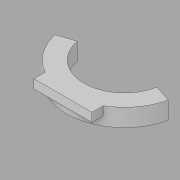
# Autodesk Inventor part: g_jaws
Saved by Autodesk Inventor 2019 (Build 230136000, 136)
## iProperties
Created: 2021-11-03
Part Number: g_jaws
Material: Generic
Document SubType Name: Modeling
Designer: Mohamed
Density: 1 g/cm^3
Appearance: Default
Author: Mohamed
Autodesk Inventor part; units mm, degrees
ref_plane "YZ Plane" through (0, 0, 0) normal (1, 0, 0) x (0, 1, 0)
ref_plane "XZ Plane" through (0, 0, 0) normal (0, 1, 0) x (-1, 0, 0)
ref_plane "XY Plane" through (0, 0, 0) normal (0, 0, 1) x (1, 0, 0)
sketch "Sketch1" plane through (0, 0, 0) normal (0, 1, 0) x (-1, 0, 0)
  line L0 (32.1869, 7.2802) -> (22.6166, 4.1818)
  line L1 (-32.1869, 7.2802) -> (-22.6166, 4.1818)
  arc A0 (32.1869, 7.2802) -> (-32.1869, 7.2802) centre (0, 0) ccw
  arc A1 (22.6166, 4.1818) -> (-22.6166, 4.1818) centre (0, 0) ccw
  dimension "d7" = 23
  dimension "d8" = 33
  constraints: 4 end point, 4 point on circle, 2 centre point, 1 coincident
  measures "d7" radius of A1
  measures "d8" radius of A0
extrude "Extrusion1" add sketch "Sketch1" along normal blind 10
sketch "Sketch2" plane through (0, 10, 0) normal (0, 1, 0) x (1, 0, 0)
  arc A0 (-32.1869, -7.2802) -> (32.1869, -7.2802) centre (0, 0) ccw projected
  line L0 (0, -35) -> (-16.5, -35)
  line L1 (-16.5, -35) -> (16.5, -35)
  line L2 (-16.5, -35) -> (-16.5, -28.5788)
  line L3 (16.5, -35) -> (16.5, -28.5788)
  dimension "d10" = 16.5
  dimension "d11" = 33
  constraints: 8 end point, 2 point on circle, 2 vertical, 1 horizontal, 1 point on line
  measures "d10" distance of L0.start L0.end
  measures "d11" distance of L0.end L1.end
extrude "Extrusion2" add sketch "Sketch2" against normal blind 5
body "Solid1"
